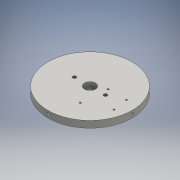
# Autodesk Inventor part: outsideCover
Saved by Autodesk Inventor 2016 (Build 200138000, 138)
## iProperties
Created: 2016-10-27
Part Number: outsideCover
Material: 一般
Document SubType Name: Modeling
Designer: Daisuke
Density: 1 g/cm^3
Appearance: 既定
Author: Daisuke
Autodesk Inventor part; units mm, degrees
ref_plane "XY Plane" through (0, 0, 0) normal (0, 0, 1) x (1, 0, 0)
sketch "スケッチ1" plane through (0, 0, 0) normal (0, 0, 1) x (1, 0, 0)
  circle A0 centre (0, 0) radius 50
  dimension "d0" = 100
  constraints: 1 centre point, 1 coincident
  measures "d0" diameter of A0
extrude "押し出し1" add sketch "スケッチ1" along normal blind 8
ref_plane "作業平面1" through (50, 0, 0) normal (1, 0, 0) x (0, 1, 0)
ref_plane "作業平面2" through (-50, 0, 0) normal (1, 0, 0) x (0, 1, 0)
ref_plane "作業平面3" through (0, 50, 0) normal (0, 1, 0) x (-1, 0, 0)
ref_plane "作業平面4" through (0, -50, 0) normal (0, 1, 0) x (-1, 0, 0)
sketch "スケッチ2" plane through (50, 0, 0) normal (1, 0, 0) x (0, 1, 0)
  line L0 (0, 0) -> (0, 4) construction
  circle A0 centre (0, 4) radius 1.5
  dimension "d7" = 4
  dimension "d8" = 3
  constraints: 2 end point, 1 centre point, 1 coincident, 1 vertical
  measures "d7" distance of L0.start L0.end
  measures "d8" diameter of A0
extrude "押し出し2" cut sketch "スケッチ2" against normal blind 5
sketch "スケッチ3" plane through (-50, 0, 0) normal (1, 0, 0) x (0, 1, 0)
  line L0 (0, 0) -> (0, 4) construction
  circle A0 centre (0, 4) radius 1.5
  dimension "d11" = 4
  dimension "d12" = 3
  constraints: 2 end point, 1 centre point, 1 coincident, 1 vertical
  measures "d11" distance of L0.start L0.end
  measures "d12" diameter of A0
extrude "押し出し3" cut sketch "スケッチ3" along normal blind 5
sketch "スケッチ4" plane through (0, 50, 0) normal (0, 1, 0) x (-1, 0, 0)
  line L0 (0, 0) -> (0, 4) construction
  circle A0 centre (0, 4) radius 1.5
  dimension "d15" = 4
  dimension "d16" = 3
  constraints: 2 end point, 1 centre point, 1 coincident, 1 vertical
  measures "d15" distance of L0.start L0.end
  measures "d16" diameter of A0
extrude "押し出し4" cut sketch "スケッチ4" against normal blind 5
sketch "スケッチ5" plane through (0, -50, 0) normal (0, 1, 0) x (-1, 0, 0)
  line L0 (0, 0) -> (0, 4) construction
  circle A0 centre (0, 4) radius 1.5
  dimension "d19" = 4
  dimension "d20" = 3
  constraints: 2 end point, 1 centre point, 1 coincident, 1 vertical
  measures "d19" distance of L0.start L0.end
  measures "d20" diameter of A0
extrude "押し出し5" cut sketch "スケッチ5" along normal blind 5
thread "ねじ1" size "M3x0.5" class "6H" standard "ANSI Metric M Profile" full length
thread "ねじ2" size "M3x0.5" class "6H" standard "ANSI Metric M Profile" full length
thread "ねじ3" size "M3x0.5" class "6H" standard "ANSI Metric M Profile" full length
thread "ねじ4" size "M3x0.5" class "6H" standard "ANSI Metric M Profile" full length
sketch "スケッチ8" plane through (0, 0, 8) normal (0, 0, 1) x (1, 0, 0)
  line L0 (0, 0) -> (18.5, 0) construction
  line L1 (0, 0) -> (-18.5, 0) construction
  circle A0 centre (18.5, 0) radius 2
  circle A1 centre (-18.5, 0) radius 2
  circle A2 centre (0, 0) radius 6.5
  dimension "d62" = 18.5
  dimension "d63" = 18.5
  dimension "d64" = 4
  dimension "d65" = 4
  dimension "d66" = 13
  constraints: 4 end point, 3 centre point, 3 coincident, 2 horizontal
  measures "d62" distance of L0.start L0.end
  measures "d63" distance of L0.start L1.end
  measures "d64" diameter of A0
  measures "d65" diameter of A1
  measures "d66" diameter of A2
extrude "押し出し7" cut sketch "スケッチ8" against normal blind 8
thread "ねじ7" size "M4x0.7" class "6H" standard "ANSI Metric M Profile" full length
thread "ねじ8" size "M4x0.7" class "6H" standard "ANSI Metric M Profile" full length
sketch "スケッチ9" plane through (0, 0, 8) normal (0, 0, 1) x (1, 0, 0)
  line L0 (0, 0) -> (25, 0) construction
  line L1 (25, 0) -> (25, -1) construction
  line L2 (25, 0) -> (25, 7.5) construction
  circle A0 centre (36, 7.5) radius 1
  line L3 (36, 7.5) -> (14, 7.5) construction
  circle A1 centre (14, 7.5) radius 1
  line L4 (25, -1) -> (25, -10) construction
  line L5 (25, -10) -> (38.5, -10) construction
  line L6 (25, -10) -> (25, -23) construction
  line L7 (25, -23) -> (11.5, -23) construction
  circle A2 centre (11.5, -23) radius 1
  circle A3 centre (38.5, -10) radius 1
  dimension "d92" = 25
  dimension "d103" = 7.5
  dimension "d105" = 2
  dimension "d107" = 22
  dimension "d108" = 2
  dimension "d109" = 17.5
  dimension "d110" = 13.5
  dimension "d112" = 13
  dimension "d113" = 13.5
  dimension "d117" = 2
  dimension "d120" = 2
  constraints: 16 end point, 4 centre point, 4 vertical, 3 coincident, 3 horizontal, 1 perpendicular
  measures "d92" distance of L0.start L0.end
  measures "d103" distance of L0.end L2.end
  measures "d105" diameter of A0
  measures "d107" distance of L3.start L3.end
  measures "d108" diameter of A1
  measures "d109" distance of L4.end L2.end
  measures "d110" distance of L5.end L4.end
  measures "d112" distance of L4.end L6.end
  measures "d113" distance of L6.end L7.end
  measures "d117" diameter of A2
  measures "d120" diameter of A3
extrude "押し出し9" cut sketch "スケッチ9" against normal blind 8
